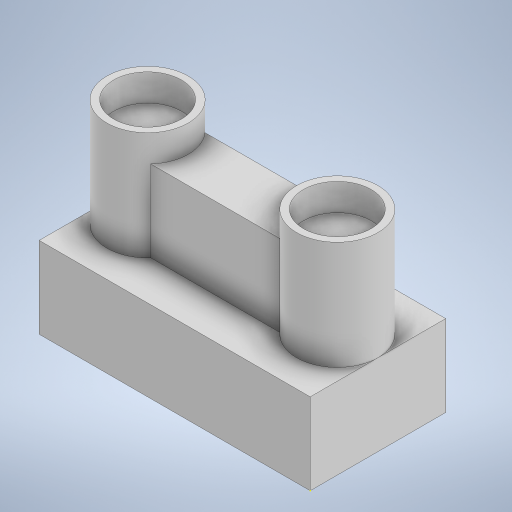
# Autodesk Inventor part: distanceSensor
Saved by Autodesk Inventor 2024.3 (Build 283343000, 343)
## iProperties
Created: 2024-11-20
Part Number: distanceSensor
Material: Generic
Document SubType Name: Modeling
Designer: Ryba
Density: 1 g/cm^3
Appearance: Default
Author: Ryba
Autodesk Inventor part; units mm, degrees
ref_plane "YZ Plane" through (0, 0, 0) normal (1, 0, 0) x (0, 1, 0)
ref_plane "XZ Plane" through (0, 0, 0) normal (0, 1, 0) x (-1, 0, 0)
ref_plane "XY Plane" through (0, 0, 0) normal (0, 0, 1) x (1, 0, 0)
sketch "Sketch1" plane through (0, 0, 0) normal (0, 1, 0) x (-1, 0, 0)
  point P0 (0, 0)
sketch "Sketch2" plane through (0, 0, 0) normal (0, 1, 0) x (-1, 0, 0)
  line L0 (0, 0) -> (10, 0)
  line L1 (10, 0) -> (10, -5)
  line L2 (10, -5) -> (0, -5)
  line L3 (0, -5) -> (0, 0)
  dimension "d0" = 10
  dimension "d1" = 5
  constraints: 8 end point, 2 parallel, 1 horizontal, 1 perpendicular
  measures "d0" distance of L1.end L2.end
  measures "d1" distance of L0.end L1.end
extrude "Extrusion1" add sketch "Sketch2" along normal blind 3
sketch "Sketch3" plane through (0, 3, 0) normal (0, 1, 0) x (1, 0, 0)
  line L0 (-10, 5) -> (-10, 0) projected
  line L1 (-10, 2.5) -> (0, 2.5)
  line L2 (-10, 2.5) -> (-8.5, 2.5)
  line L3 (0, 2.5) -> (-1.5, 2.5)
  circle A0 centre (-8.5, 2.5) radius 1.5
  circle A1 centre (-1.5, 2.5) radius 1.5
  line L4 (0, 0) -> (0, 5) projected
  line L5 (-7.382, 1.5) -> (-2.618, 1.5)
  line L6 (-2.618, 3.5) -> (-7.382, 3.5)
  constraints: 10 end point, 4 point on circle, 2 centre point, 2 coincident, 2 perpendicular, 2 point on line, 1 horizontal, 1 midpoint
extrude "Extrusion2" add sketch "Sketch3" along normal blind 4
sketch "Sketch4" plane through (0, 7, 0) normal (0, 1, 0) x (1, 0, 0)
  arc A0 (-10, 2.5) -> (-7.382, 1.5) centre (-8.5, 2.5) ccw projected
  circle A1 centre (-8.5, 2.5) radius 1.25
  arc A2 (-2.618, 1.5) -> (-2.618, 3.5) centre (-1.5, 2.5) ccw projected
  circle A3 centre (-1.5, 2.5) radius 1.25
  arc A4 (-2.618, 3.5) -> (-2.618, 1.5) centre (-1.5, 2.5) ccw
  arc A5 (-7.382, 1.5) -> (-7.382, 3.5) centre (-8.5, 2.5) ccw
  line L0 (-7.382, 1.5) -> (-2.618, 1.5)
  line L1 (-7.382, 3.5) -> (-2.618, 3.5)
  point P0 (0, 0)
  constraints: 4 centre point, 4 coincident, 4 end point, 4 point on circle, 2 horizontal
extrude "Extrusion3" cut sketch "Sketch4" against normal blind 1 contours A1 | L0 A5 L1 A4 | A3
sketch "Sketch5" plane through (0, 0, 0) normal (0, -1, 0) x (1, 0, 0)
  line L0 (0, -5) -> (-10, -5) projected
  line L1 (0, -5) -> (-2, -5)
  line L2 (-10, -5) -> (-8, -5)
  line L3 (-2, -5) -> (-1.5, -5)
  line L4 (-1.5, -5) -> (-1.5, -5.5)
  line L5 (-2.5, -5.5) -> (-2.5, -5)
  line L6 (-2.5, -5) -> (-2, -5)
  line L7 (-8, -5) -> (-8.5, -5)
  line L8 (-8.5, -5) -> (-8.5, -5.5)
  line L9 (-7.5, -5.5) -> (-7.5, -5)
  line L10 (-7.5, -5) -> (-8, -5)
  arc A0 (-2.5, -5.5) -> (-1.5, -5.5) centre (-2, -5.5) ccw
  arc A1 (-8.5, -5.5) -> (-7.5, -5.5) centre (-8, -5.5) ccw
  point P0 (0, 0)
  dimension "d19" = 2
  constraints: 20 end point, 6 point on line, 4 perpendicular, 4 point on circle, 2 centre point, 1 collinear, 1 horizontal
  measures "d19" distance of L0.end L2.end
extrude "Extrusion4" add sketch "Sketch5" against normal blind 0.3
sketch "Sketch6" plane through (0, 0.3, 0) normal (0, 1, 0) x (1, 0, 0)
  arc A0 (-1.5, 5.5) -> (-2.5, 5.5) centre (-2, 5.5) ccw projected
  circle A1 centre (-2, 5.5) radius 0.4
  arc A2 (-7.5, 5.5) -> (-8.5, 5.5) centre (-8, 5.5) ccw projected
  circle A3 centre (-8, 5.5) radius 0.4
  point P0 (0, 0)
  dimension "d30" = 0.8
  dimension "d31" = 0.8
  constraints: 2 centre point, 2 coincident
  measures "d30" diameter of A1
  measures "d31" diameter of A3
extrude "Extrusion5" cut sketch "Sketch6" against normal blind 0.3
thread "Thread1" size "M0.3x0.08" class "6H" standard "ISO Metric profile" full length
thread "Thread2" size "M0.3x0.08" class "6H" standard "ANSI Metric M Profile" full length
body "Solid1"
